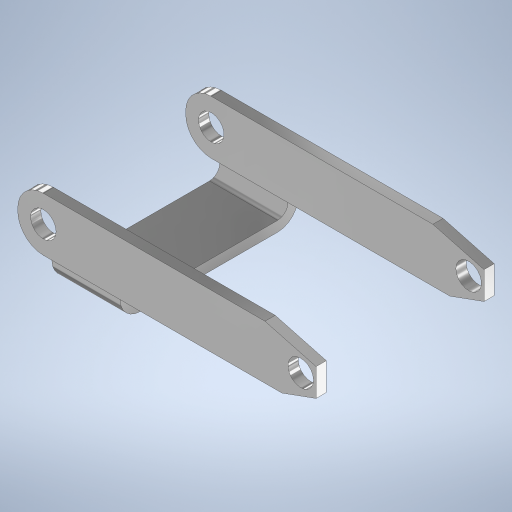
# Autodesk Inventor part: Lever 1
Saved by Autodesk Inventor 2024 (Build 280153000, 153)
## iProperties
Created: 2007-06-22
Part Number: Lever 1
Material: Steel
Document SubType Name: Sheet Metal
Designer: G.K.
Description: Lever 1
Mass: 5.30882 g
Surface Area: 13.9122 cm^2
Volume: 0.676283 cm^3
Density: 7.85 g/cm^3
Sheet Metal Rule: Default
Appearance: Chrome - Polished
Mase: 0.00530882
Autodesk Inventor part; units mm, degrees
ref_plane "YZ Plane" through (0, 0, 0) normal (1, 0, 0) x (0, 1, 0)
ref_plane "XZ Plane" through (0, 0, 0) normal (0, 1, 0) x (-1, 0, 0)
ref_plane "XY Plane" through (0, 0, 0) normal (0, 0, 1) x (1, 0, 0)
sketch "Sketch1" plane through (0, 0, 0) normal (0, 0, 1) x (1, 0, 0)
  line L0 (-4, 9.25) -> (4, 9.25)
  line L1 (4, 9.25) -> (4, -9.25)
  line L2 (4, -9.25) -> (-4, -9.25)
  line L3 (-4, -9.25) -> (-4, 9.25)
  point P0 (0, 0)
  point P1 (-4, 0)
  point P2 (0, -9.25)
  dimension "d0" = 18.5
  dimension "d1" = 8
  constraints: 8 end point, 2 midpoint, 2 parallel, 1 horizontal, 1 horizontal alignment, 1 perpendicular, 1 vertical alignment
  measures "d0" distance of L2.end L0.start
  measures "d1" distance between parallel lines of L1 L3
extrude "Plate1" add sketch "Sketch1" along normal blind 1.2
sketch "Sketch2" plane through (4, -9.25, 1.2) normal (0, 1, 0) x (-1, 0, 0)
  line L0 (0, 0) -> (8, 0)
  line L1 (8, 0) -> (8, 7.5)
  line L2 (8, 7.5) -> (0, 7.5)
  line L3 (0, 7.5) -> (0, 0)
  constraints: 4 end point, 4 other
sheet face with bend "Flange1" sketch "Sketch2" thickness 1.2 toward (0, -1, 0) bend radius 1.2 relief straight relief width 1.2 relief depth 0.6
bend "Bend1"
sketch "Sketch3" plane through (-4, 9.25, 1.2) normal (0, -1, 0) x (1, 0, 0)
  line L0 (0, 0) -> (8, 0)
  line L1 (8, 0) -> (8, 7.5)
  line L2 (8, 7.5) -> (0, 7.5)
  line L3 (0, 7.5) -> (0, 0)
  constraints: 4 end point, 4 other
sheet face with bend "Flange2" sketch "Sketch3" thickness 1.2 toward (0, 1, 0) bend radius 1.2 relief straight relief width 1.2 relief depth 0.6
bend "Bend2"
sketch "Sketch5" plane through (-4, -10.45, 8.7) normal (0, -1, 0) x (1, 0, 0)
  line L0 (0, -6.3) -> (0, 0) projected
  line L1 (8, 0) -> (31, 0)
  line L2 (31, 0) -> (31, -6.3)
  line L3 (31, -6.3) -> (8, -6.3)
  line L4 (8, -6.3) -> (8, 0)
  line L5 (0, 0) -> (-1, 0)
  line L6 (-4, -3) -> (-4, -3.3)
  line L7 (-1, -6.3) -> (0, -6.3)
  line L8 (0, -6.3) -> (0, 0)
  arc A0 (-1, 0) -> (-4, -3) centre (-1, -3) ccw
  arc A1 (-4, -3.3) -> (-1, -6.3) centre (-1, -3.3) ccw
  point P0 (4, -8.7)
  dimension "d18" = 6.3
  dimension "d19" = 4
  dimension "d20" = 35
  dimension "d21" = 3
  constraints: 16 end point, 4 parallel, 4 point on circle, 4 tangent, 2 centre point, 2 horizontal, 2 perpendicular, 1 collinear, 1 equal radius
  measures "d18" distance between parallel lines of L3 L1
  measures "d19" distance between parallel lines of L0 L6
  measures "d20" distance between parallel lines of L2 L6
  measures "d21" radius of A0
sheet face with bend "Face2" sketch "Sketch5" thickness 1.2 toward (0, 1, 0) bend radius 1.2 relief straight relief width 1.2 relief depth 0.6
bend "Bend3"
sketch "Sketch6" plane through (4, -10.45, 2.4) normal (0, -1, 0) x (1, 0, 0)
  line L0 (0, 0) -> (23, 0) projected
  line L1 (23, 0) -> (23, 6.3) projected
  line L2 (23, 6.3) -> (-9, 6.3) projected
  line L3 (19, 0) -> (23, 1.4559)
  line L4 (23, 4.6923) -> (17, 6.3)
  point P0 (-4, -2.4)
  dimension "d27" = 20
  dimension "d28" = 15
  dimension "d29" = 4
  dimension "d30" = 6
  constraints: 4 end point, 4 point on line
  measures "d27" angle of L0 L3
  measures "d28" angle of L4 L2
  measures "d29" distance from line of L3.start L1
  measures "d30" horizontal distance of L4.start L4.end
extrude "Cut1" cut sketch "Sketch6" against normal blind 1.2
mirror "Mirror1" about plane through (0, 0, 0) normal (0, 1, 0) of "Face2", "Cut1"
sketch "Sketch8" plane through (-5, -10.45, 2.4) normal (0, -1, 0) x (1, 0, 0)
  circle A0 centre (30.1983, 3.1495) radius 1.5
  circle A1 centre (0, 3.15) radius 1.5
  line L0 (0, 3.15) -> (30.1983, 3.1495)
  point P0 (5, -2.4)
  constraints: 2 centre point, 2 end point, 4 other
hole "Hole2" at (25.1983, -10.45, 5.5495) at (-5, -10.45, 5.55) direction (0, 1, 0) diameter 3 depth 22 tip angle 118
equation "\"d31\" = Thickness"
equation "\"d50\" = Thickness"
equation "\"d3\" = BendReliefWidth"
equation "\"d5\" = MinimumRemnant"
equation "\"d9\" = BendRadius"
equation "\"d4\" = BendReliefDepth"
equation "\"d6\" = BendRadius"
equation "\"d10\" = BendReliefWidth"
equation "\"d12\" = MinimumRemnant"
equation "\"d16\" = BendRadius"
equation "\"d11\" = BendReliefDepth"
equation "\"d13\" = BendRadius"
equation "\"d22\" = BendRadius"
equation "\"d23\" = BendReliefWidth"
equation "\"d25\" = MinimumRemnant"
equation "\"d24\" = BendReliefDepth"
equation "\"d26\" = BendRadius"
equation "\"BendRadius\" = Thickness"
equation "\"BendReliefWidth\" = Thickness"
equation "\"BendReliefDepth\" = 0.5 * Thickness"
equation "\"CornerReliefSize\" = 4 * Thickness"
equation "\"MinimumRemnant\" = 2 * Thickness"
equation "\"TransitionRadius\" = BendRadius"
equation "\"d2\" = BendRadius"
equation "\"JacobiRadiusSize\" = Thickness"
equation "\"GapSize\" = Thickness"
equation "\"Thickness\" = 1.2"
body "Solid1"
